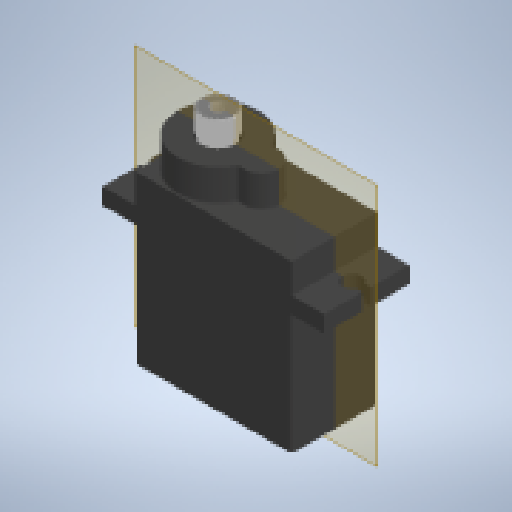
# Autodesk Inventor part: MG90S Servo Motor
Saved by Autodesk Inventor 2023 (Build 270158000, 158)
## iProperties
Created: 2020-02-24
Part Number: MG90S Servo Motor
Material: Generic
Document SubType Name: Modeling
Designer: DELL
Density: 1 g/cm^3
Appearance: Ducati - Light Black
Author: DELL
Autodesk Inventor part; units mm, degrees
ref_plane "YZ Plane" through (0, 0, 0) normal (1, 0, 0) x (0, 1, 0)
ref_plane "XZ Plane" through (0, 0, 0) normal (0, 1, 0) x (-1, 0, 0)
ref_plane "XY Plane" through (0, 0, 0) normal (0, 0, 1) x (1, 0, 0)
sketch "Sketch1" plane through (0, 0, 0) normal (0, 0, 1) x (1, 0, 0)
  line L0 (-16.1, 17.5) -> (-11.4, 17.5)
  line L1 (-11.4, 19.9) -> (-16.1, 19.9)
  line L2 (-11.4, 19.9) -> (-11.4, 24.2)
  line L3 (-11.4, 24.2) -> (11.4, 24.2)
  line L4 (16.1, 19.9) -> (16.1, 17.5)
  line L5 (11.4, 0) -> (11.4, 17.5)
  line L6 (-11.4, 17.5) -> (-11.4, 0)
  line L7 (11.4, 0) -> (-11.4, 0)
  line L8 (11.4, 17.5) -> (16.1, 17.5)
  line L9 (-16.1, 17.5) -> (-16.1, 19.9)
  line L10 (11.4, 24.2) -> (11.4, 19.9)
  line L11 (11.4, 19.9) -> (16.1, 19.9)
  point P0 (0, 0)
  point P1 (0, 0)
  point P2 (0, 24.2)
  dimension "d5" = 4.7
  dimension "d6" = 2.4
  dimension "d7" = 17.5
  dimension "d8" = 22.8
  dimension "d20" = 4.3
  dimension "d21" = 4.7
  dimension "d89" = 32.2
  constraints: 24 end point, 4 equal length, 4 horizontal, 2 collinear, 2 midpoint, 2 parallel, 2 perpendicular, 2 vertical, 1 coincident, 1 vertical alignment
  measures "d5" distance of L0.start L0.end
  measures "d6" distance of L4.start L4.end
  measures "d7" distance of L5.start L5.end
  measures "d8" distance of L2.end L3.end
  measures "d20" distance of L1.start L2.end
  measures "d21" distance of L5.end L4.end
  measures "d89" distance of L4.end L0.start
extrude "Extrusion1" add sketch "Sketch1" along normal mid plane 12.4
sketch "Sketch2" plane through (-11.4, 24.2, 6.2) normal (0, 1, 0) x (1, 0, 0)
  circle A0 centre (5.9, 6.2) radius 2.55
  arc A1 (11.2442, 8.7) -> (11.2442, 3.7) centre (5.9, 6.2) ccw
  line L0 (12.2, 8.7) -> (11.2442, 8.7)
  arc A2 (12.2, 3.7) -> (12.2, 8.7) centre (12.2, 6.2) ccw
  line L1 (11.2442, 3.7) -> (12.2, 3.7)
  line L2 (0, 12.4) -> (0, 0) construction
  line L3 (-11.14, 6.2) -> (33.94, 6.2) construction
  point P0 (11.4, 6.2)
  dimension "d13" = 5.9
  dimension "d14" = 2.5
  dimension "d15" = 6.3
  dimension "d16" = 5.1
  dimension "d17" = 0.9558
  constraints: 4 end point, 4 point on circle, 3 centre point, 3 tangent, 2 point on line, 1 concentric, 1 parallel
  measures "d13" radius of A1
  measures "d14" radius of A2
  measures "d15" distance of A2.centre A0.centre
  measures "d16" diameter of A0
  measures "d17" distance of L0.start L0.end
extrude "Extrusion2" add sketch "Sketch2" along normal blind 4.5
sketch "Sketch3" plane through (11.4, 19.9, 6.2) normal (0, 1, 0) x (1, 0, 0)
  line L0 (0, 12.4) -> (0, 0) construction
  line L1 (4.7, 12.4) -> (4.7, 0) construction
  line L2 (0, 6.2) -> (4.7, 6.2) construction
  point P0 (-11.4, 6.2)
  point P1 (2.6, 6.2)
  dimension "d86" = 2.1
  constraints: 2 end point, 2 midpoint, 1 point on line
  measures "d86" distance of point (2.6, 6.2) L2.end
hole "Hole1" at (14, 19.9, 0) direction (0, -1, 0) diameter 2.75 depth 8 tip angle 118
sketch "Sketch4" plane through (11.4, 19.9, 6.2) normal (0, 1, 0) x (1, 0, 0)
  circle A0 centre (2.6, 6.2) radius 1.375 construction
  line L0 (3.8372, 6.8) -> (4.7, 6.8)
  line L1 (3.8372, 5.6) -> (4.7, 5.6)
  line L2 (4.7, 12.4) -> (4.7, 0) construction
  line L3 (4.7, 5.6) -> (4.7, 6.8)
  arc A1 (3.8372, 5.6) -> (3.8372, 6.8) centre (2.6, 6.2) ccw
  point P0 (-11.4, 6.2)
  dimension "d31" = 1.2
  dimension "d34" = 0.6
  constraints: 6 end point, 4 point on circle, 2 collinear, 1 centre point, 1 coincident, 1 horizontal
  measures "d31" distance between parallel lines of L1 L0
  measures "d34" vertical distance of A1.centre L0.start
extrude "Extrusion3" cut sketch "Sketch4" against normal through all
mirror "Mirror1" about plane through (0, 0, 0) normal (1, 0, 0) of "Hole1", "Extrusion3"
fillet "Fillet1" radius 0.2 5 edges at (3.3, 24.2, 0) (0.3221, 24.2, -2.5) (0.3221, 24.2, 2.5) (-6.7805, 24.2, 5.7594) (-6.7805, 24.2, -5.7594)
fillet "Fillet2" radius 0.4 4 edges at (11.4, 8.75, 6.2) (11.4, 8.75, -6.2) (-11.4, 8.75, -6.2) (-11.4, 8.75, 6.2)
sketch "Sketch5" plane through (-11.4, 28.7, 6.2) normal (0, 1, 0) x (1, 0, 0)
  circle A0 centre (5.9, 6.2) radius 2.55 construction
  circle A1 centre (5.9, 6.2) radius 2.1835
  point P0 (11.4, 6.2)
  dimension "d39" = 4.367
  constraints: 1 centre point, 1 coincident
  measures "d39" diameter of A1
extrude "Extrusion4" add sketch "Sketch5" along normal blind 3.5 and the other way blind 10 separate body
sketch "Sketch6" plane through (-5.5, 32.2, 0) normal (0, 1, 0) x (1, 0, 0)
  arc A0 (0.1023, 2.4729) -> (-0.1023, 2.4729) centre (0, 0) ccw
  spline S0 degree 4 poles (0.2432, 2.2369) (0.2144, 2.3003) (0.181, 2.3617) (0.1436, 2.4199) (0.1023, 2.4729) knots 0 0 0 0 0 1 1 1 1 1
  spline S1 degree 4 poles (-0.1023, 2.4729) (-0.1425, 2.4203) (-0.1793, 2.3624) (-0.2129, 2.3009) (-0.2432, 2.2369) knots 0 0 0 0 0 1 1 1 1 1
  arc A1 (-0.2432, 2.2369) -> (-0.2576, 2.2014) centre (0.6912, 1.8392) ccw
  arc A2 (-0.3072, 2.1618) -> (-0.2576, 2.2014) centre (-0.316, 2.2237) ccw
  arc A3 (0.2576, 2.2014) -> (0.2432, 2.2369) centre (-0.6912, 1.8392) ccw
  arc A4 (0.2576, 2.2014) -> (0.3072, 2.1618) centre (0.316, 2.2237) ccw
  arc A5 (0.3072, 2.1618) -> (-0.3072, 2.1618) centre (0, 0) ccw
  circle A6 centre (0, 0) radius 2.1835 construction
  point P0 (0.2123, 2.3002)
  point P1 (0.1783, 2.3611)
  point P2 (0.1415, 2.419)
  point P3 (-0.1402, 2.4199)
  point P4 (-0.1765, 2.3626)
  point P5 (-0.2109, 2.3013)
  dimension "d50" = 2.475
  dimension "d51" = 2.4729
  dimension "d52" = 0.1023
  dimension "d53" = 2.2237
  dimension "d55" = 0.316
  dimension "d56" = 0.316
  dimension "d57" = 0.0625
  dimension "d58" = 1.0155
  dimension "d59" = 1.8392
  dimension "d60" = 0.6912
  dimension "d61" = 1.3823
  dimension "d62" = 1.0155
  constraints: 14 point on circle, 6 centre point, 2 concentric, 2 horizontal alignment, 1 coincident, 1 equal radius, 10 other
  measures "d50" radius of A0
  measures "d51" vertical distance of A0.end A0.centre
  measures "d52" horizontal distance of A0.end A0.centre
  measures "d53" vertical distance of A2.centre A0.centre
  measures "d55" horizontal distance of A4.centre A5.centre
  measures "d56" horizontal distance of A2.centre A0.centre
  measures "d57" radius of A4
  measures "d58" radius of A1
  measures "d59" vertical distance of A1.centre A0.centre
  measures "d60" horizontal distance of A1.centre A0.centre
  measures "d61" distance of A1.centre A3.centre
  measures "d62" radius of A3
extrude "Extrusion5" add sketch "Sketch6" against normal blind 3 bodies 1
pattern_circular "Circular Pattern1" count 20 over 360 about axis through (-5.5, 28.7, 0) along (0, 1, 0) of "Extrusion5" bodies 1
chamfer "Chamfer2" distance 0.15 angle 45 20 edges at (-4.0452, 32.2, 2.0023) (-3.4977, 32.2, 1.4548) (-3.1461, 32.2, 0.7648) (-3.025, 32.2, 0) (-3.1461, 32.2, -0.7648) (-3.4977, 32.2, -1.4548) (-4.0452, 32.2, -2.0023) (-4.7352, 32.2, -2.3539) (-5.5, 32.2, -2.475) (-6.2648, 32.2, -2.3539) (-6.9548, 32.2, -2.0023) (-7.5023, 32.2, -1.4548) (-7.8539, 32.2, -0.7648) (-7.975, 32.2, 0) (-7.8539, 32.2, 0.7648) (-7.5023, 32.2, 1.4548) (-6.9548, 32.2, 2.0023) (-6.2648, 32.2, 2.3539) (-5.5, 32.2, 2.475) (-4.7352, 32.2, 2.3539)
sketch "Sketch7" plane through (-5.5, 32.2, 0) normal (0, 1, 0) x (1, 0, 0)
  circle A0 centre (0, 0) radius 2.55 construction
  point P0 (5.5, 0)
  constraints: 1 coincident
hole "Hole2" at (-5.5, 32.2, 0) direction (0, -1, 0) diameter 2.013 depth 8 tip angle 118 bodies 2 thread size "M2.5x0.45" class "6H" standard "ANSI Metric M Profile"
sketch "Ref Sketch" plane through (-11.4, 28.7, 6.2) normal (0, 1, 0) x (1, 0, 0)
  line L0 (0, 4.6508) -> (0, 0) construction
  line L1 (22.8, 12.4) -> (22.8, 0) construction
  circle A0 centre (5.9, 6.2) radius 1.0065 construction
  line L2 (22.8, 12.4) -> (0, 0) construction
  arc A1 (-3.8372, 5.6) -> (-3.8372, 6.8) centre (-2.6, 6.2) ccw projected
  arc A2 (26.6372, 6.8) -> (26.6372, 5.6) centre (25.4, 6.2) ccw projected
  line L3 (0, 12.4) -> (22.8, 12.4) projected
  line L4 (0, 12.4) -> (0, 7.7492) projected
  line L5 (22.8, 0) -> (0, 0) projected
  point P0 (11.4, 6.2)
  point P1 (11.4, 6.2)
  dimension "d78" = 16.9
  dimension "d79" = 5.9
  dimension "d80" = 5.5
  dimension "d81" = 28
  dimension "d87" = 22.8
  dimension "d88" = 12.4
  constraints: 2 end point, 1 coincident
  measures "d78" horizontal distance of A0.centre L1.end
  measures "d79" horizontal distance of A0.centre L0.end
  measures "d80" distance of point (11.4, 6.2) A0.centre
  measures "d81" distance of A2.centre A1.centre
  measures "d87" distance of L1.start L3.start
  measures "d88" distance of L1.end L1.start
ref_plane "Work Plane2" through (0, 0, 0) normal (0, 0, 1) x (1, 0, 0)
body "Solid1"
body "Solid2"
